Autodesk Fusion 360 part; units mm, degrees
(part 4 of 5)
  spline S14 degree 5 poles (-118.7463, -28.9627) (-118.7429, -28.9568) (-118.7364, -28.9449) (-118.7271, -28.9268) (-118.7157, -28.9022) (-118.7027, -28.8708) (-118.6906, -28.8389) (-118.6791, -28.8067) (-118.668, -28.7744) (-118.657, -28.7419) (-118.6463, -28.7093) (-118.6358, -28.6766) (-118.6257, -28.6437) (-118.6161, -28.6105) (-118.607, -28.5772) (-118.5983, -28.5436) (-118.59, -28.5099) (-118.582, -28.476) (-118.5742, -28.4421) (-118.5667, -28.408) (-118.5595, -28.3737) (-118.5526, -28.3394) (-118.5459, -28.305) (-118.5395, -28.2704) (-118.5334, -28.2357) (-118.5276, -28.2008) (-118.5221, -28.1659) (-118.5168, -28.1309) (-118.5118, -28.0957) (-118.507, -28.0605) (-118.5025, -28.0252) (-118.4982, -27.9897) (-118.4942, -27.9542) (-118.4904, -27.9186) (-118.4868, -27.8829) (-118.4835, -27.8471) (-118.4804, -27.8113) (-118.4775, -27.7753) (-118.4749, -27.7393) (-118.4725, -27.7032) (-118.4703, -27.667) (-118.4684, -27.6307) (-118.4666, -27.5944) (-118.4651, -27.558) (-118.4638, -27.5215) (-118.4627, -27.4849) (-118.4618, -27.4483) (-118.4612, -27.4116) (-118.4607, -27.3749) (-118.4605, -27.3381) (-118.4604, -27.3012) (-118.4606, -27.2643) (-118.461, -27.2273) (-118.4616, -27.1902) (-118.4624, -27.1531) (-118.4634, -27.1159) (-118.4646, -27.0787) (-118.466, -27.0414) (-118.4676, -27.0041) (-118.4694, -26.9667) (-118.4714, -26.9293) (-118.4736, -26.8918) (-118.476, -26.8542) (-118.4785, -26.8167) (-118.4813, -26.779) (-118.4843, -26.7414) (-118.4875, -26.7036) (-118.4908, -26.6659) (-118.4944, -26.6281) (-118.4981, -26.5902) (-118.5021, -26.5523) (-118.5053, -26.522) (-118.5079, -26.4992) (-118.5097, -26.484) (-118.5105, -26.4764) knots 0 0 0 0 0 0 0.01428571 0.02857143 0.04285714 0.05714286 0.07142857 0.08571429 0.1 0.11428571 0.12857143 0.14285714 0.15714286 0.17142857 0.18571429 0.2 0.21428571 0.22857143 0.24285714 0.25714286 0.27142857 0.28571429 0.3 0.31428571 0.32857143 0.34285714 0.35714286 0.37142857 0.38571429 0.4 0.41428571 0.42857143 0.44285714 0.45714286 0.47142857 0.48571429 0.5 0.51428571 0.52857143 0.54285714 0.55714286 0.57142857 0.58571429 0.6 0.61428571 0.62857143 0.64285714 0.65714286 0.67142857 0.68571429 0.7 0.71428571 0.72857143 0.74285714 0.75714286 0.77142857 0.78571429 0.8 0.81428571 0.82857143 0.84285714 0.85714286 0.87142857 0.88571429 0.9 0.91428571 0.92857143 0.94285714 0.95714286 0.97142857 0.98571429 1 1 1 1 1 1
  arc A29 (-118.5105, -26.4764) -> (-119.3694, -26.0969) centre (-125, -40) ccw
  spline S15 degree 5 poles (-121.0491, -27.9451) (-121.047, -27.9386) (-121.0426, -27.9258) (-121.0354, -27.9067) (-121.025, -27.8817) (-121.0105, -27.8509) (-120.995, -27.8206) (-120.979, -27.7904) (-120.9626, -27.7604) (-120.9459, -27.7304) (-120.9291, -27.7005) (-120.9119, -27.6708) (-120.8943, -27.6412) (-120.8763, -27.6118) (-120.8578, -27.5825) (-120.8388, -27.5535) (-120.8195, -27.5247) (-120.7999, -27.4959) (-120.78, -27.4673) (-120.7598, -27.4388) (-120.7393, -27.4105) (-120.7186, -27.3822) (-120.6977, -27.3541) (-120.6764, -27.3261) (-120.6548, -27.2982) (-120.633, -27.2705) (-120.6109, -27.2429) (-120.5885, -27.2154) (-120.5659, -27.188) (-120.543, -27.1608) (-120.52, -27.1336) (-120.4967, -27.1066) (-120.4731, -27.0797) (-120.4494, -27.0529) (-120.4254, -27.0263) (-120.4011, -26.9997) (-120.3767, -26.9733) (-120.352, -26.947) (-120.3272, -26.9208) (-120.3021, -26.8947) (-120.2768, -26.8687) (-120.2513, -26.8428) (-120.2256, -26.8171) (-120.1997, -26.7914) (-120.1736, -26.7659) (-120.1473, -26.7405) (-120.1208, -26.7152) (-120.0942, -26.69) (-120.0673, -26.6649) (-120.0402, -26.64) (-120.013, -26.6151) (-119.9856, -26.5904) (-119.9579, -26.5658) (-119.9301, -26.5412) (-119.9022, -26.5168) (-119.874, -26.4926) (-119.8457, -26.4684) (-119.8172, -26.4443) (-119.7885, -26.4204) (-119.7596, -26.3965) (-119.7306, -26.3728) (-119.7014, -26.3492) (-119.6721, -26.3257) (-119.6425, -26.3023) (-119.6128, -26.279) (-119.583, -26.2558) (-119.553, -26.2328) (-119.5228, -26.2099) (-119.4924, -26.187) (-119.4619, -26.1643) (-119.4313, -26.1417) (-119.4066, -26.1237) (-119.388, -26.1103) (-119.3756, -26.1014) (-119.3694, -26.0969) knots 0 0 0 0 0 0 0.01428571 0.02857143 0.04285714 0.05714286 0.07142857 0.08571429 0.1 0.11428571 0.12857143 0.14285714 0.15714286 0.17142857 0.18571429 0.2 0.21428571 0.22857143 0.24285714 0.25714286 0.27142857 0.28571429 0.3 0.31428571 0.32857143 0.34285714 0.35714286 0.37142857 0.38571429 0.4 0.41428571 0.42857143 0.44285714 0.45714286 0.47142857 0.48571429 0.5 0.51428571 0.52857143 0.54285714 0.55714286 0.57142857 0.58571429 0.6 0.61428571 0.62857143 0.64285714 0.65714286 0.67142857 0.68571429 0.7 0.71428571 0.72857143 0.74285714 0.75714286 0.77142857 0.78571429 0.8 0.81428571 0.82857143 0.84285714 0.85714286 0.87142857 0.88571429 0.9 0.91428571 0.92857143 0.94285714 0.95714286 0.97142857 0.98571429 1 1 1 1 1 1
  line L15 (-121.0491, -27.9451) -> (-121.1835, -28.3552)
  arc A30 (-121.7948, -28.6805) -> (-121.1835, -28.3552) centre (-121.6586, -28.1994) ccw
  arc A31 (-121.7948, -28.6805) -> (-122.5797, -28.4872) centre (-125, -40) ccw
  arc A32 (-122.9699, -27.915) -> (-122.5797, -28.4872) centre (-122.4768, -27.9979) ccw
  line L16 (-122.9699, -27.915) -> (-122.8984, -27.4894)
  spline S16 degree 5 poles (-122.8984, -27.4894) (-122.8973, -27.4827) (-122.8952, -27.4693) (-122.8927, -27.4491) (-122.8903, -27.4221) (-122.8889, -27.3881) (-122.8884, -27.3541) (-122.8887, -27.3199) (-122.8892, -27.2857) (-122.89, -27.2514) (-122.8911, -27.2171) (-122.8924, -27.1828) (-122.8943, -27.1484) (-122.8966, -27.114) (-122.8994, -27.0795) (-122.9027, -27.045) (-122.9064, -27.0105) (-122.9104, -26.9759) (-122.9148, -26.9413) (-122.9194, -26.9067) (-122.9243, -26.8721) (-122.9295, -26.8375) (-122.9351, -26.8028) (-122.9409, -26.7681) (-122.9471, -26.7334) (-122.9535, -26.6987) (-122.9603, -26.664) (-122.9673, -26.6293) (-122.9746, -26.5946) (-122.9822, -26.5598) (-122.99, -26.5251) (-122.9981, -26.4903) (-123.0064, -26.4556) (-123.015, -26.4208) (-123.0239, -26.386) (-123.033, -26.3513) (-123.0424, -26.3165) (-123.052, -26.2817) (-123.0618, -26.247) (-123.0719, -26.2122) (-123.0822, -26.1775) (-123.0928, -26.1427) (-123.1036, -26.108) (-123.1146, -26.0733) (-123.1259, -26.0385) (-123.1373, -26.0038) (-123.1491, -25.9691) (-123.161, -25.9344) (-123.1731, -25.8997) (-123.1855, -25.865) (-123.1981, -25.8304) (-123.2109, -25.7957) (-123.2239, -25.7611) (-123.2371, -25.7265) (-123.2506, -25.6919) (-123.2642, -25.6573) (-123.2781, -25.6227) (-123.2921, -25.5882) (-123.3064, -25.5536) (-123.3209, -25.5191) (-123.3356, -25.4846) (-123.3504, -25.4501) (-123.3655, -25.4157) (-123.3808, -25.3812) (-123.3963, -25.3468) (-123.412, -25.3125) (-123.4278, -25.2781) (-123.4439, -25.2438) (-123.4602, -25.2094) (-123.4766, -25.1752) (-123.4933, -25.1409) (-123.5068, -25.1135) (-123.517, -25.093) (-123.5238, -25.0793) (-123.5272, -25.0725) knots 0 0 0 0 0 0 0.01428571 0.02857143 0.04285714 0.05714286 0.07142857 0.08571429 0.1 0.11428571 0.12857143 0.14285714 0.15714286 0.17142857 0.18571429 0.2 0.21428571 0.22857143 0.24285714 0.25714286 0.27142857 0.28571429 0.3 0.31428571 0.32857143 0.34285714 0.35714286 0.37142857 0.38571429 0.4 0.41428571 0.42857143 0.44285714 0.45714286 0.47142857 0.48571429 0.5 0.51428571 0.52857143 0.54285714 0.55714286 0.57142857 0.58571429 0.6 0.61428571 0.62857143 0.64285714 0.65714286 0.67142857 0.68571429 0.7 0.71428571 0.72857143 0.74285714 0.75714286 0.77142857 0.78571429 0.8 0.81428571 0.82857143 0.84285714 0.85714286 0.87142857 0.88571429 0.9 0.91428571 0.92857143 0.94285714 0.95714286 0.97142857 0.98571429 1 1 1 1 1 1
  arc A33 (-123.5272, -25.0725) -> (-124.4641, -25.0096) centre (-125, -40) ccw
  spline S17 degree 5 poles (-125.4104, -27.3208) (-125.4106, -27.314) (-125.4109, -27.3004) (-125.4107, -27.2801) (-125.4094, -27.253) (-125.4063, -27.2191) (-125.4022, -27.1853) (-125.3974, -27.1515) (-125.3923, -27.1176) (-125.3869, -27.0838) (-125.3813, -27.0499) (-125.3753, -27.0161) (-125.3689, -26.9823) (-125.362, -26.9485) (-125.3546, -26.9147) (-125.3467, -26.8809) (-125.3385, -26.8472) (-125.3298, -26.8135) (-125.3209, -26.7798) (-125.3117, -26.7461) (-125.3022, -26.7125) (-125.2924, -26.6788) (-125.2823, -26.6452) (-125.2719, -26.6116) (-125.2611, -26.5781) (-125.2501, -26.5446) (-125.2387, -26.511) (-125.2271, -26.4776) (-125.2153, -26.4441) (-125.2031, -26.4107) (-125.1907, -26.3773) (-125.1781, -26.344) (-125.1651, -26.3106) (-125.152, -26.2773) (-125.1385, -26.2441) (-125.1249, -26.2108) (-125.1109, -26.1776) (-125.0968, -26.1445) (-125.0823, -26.1113) (-125.0677, -26.0782) (-125.0528, -26.0452) (-125.0377, -26.0121) (-125.0224, -25.9792) (-125.0068, -25.9462) (-124.991, -25.9133) (-124.975, -25.8804) (-124.9588, -25.8476) (-124.9423, -25.8148) (-124.9256, -25.7821) (-124.9087, -25.7493) (-124.8916, -25.7167) (-124.8743, -25.684) (-124.8568, -25.6515) (-124.8391, -25.6189) (-124.8211, -25.5864) (-124.803, -25.554) (-124.7846, -25.5216) (-124.7661, -25.4892) (-124.7473, -25.4569) (-124.7283, -25.4246) (-124.7092, -25.3924) (-124.6898, -25.3602) (-124.6703, -25.3281) (-124.6505, -25.296) (-124.6306, -25.264) (-124.6104, -25.232) (-124.5901, -25.2001) (-124.5696, -25.1682) (-124.5489, -25.1364) (-124.528, -25.1046) (-124.5069, -25.0729) (-124.4899, -25.0475) (-124.477, -25.0285) (-124.4684, -25.0159) (-124.4641, -25.0096) knots 0 0 0 0 0 0 0.01428571 0.02857143 0.04285714 0.05714286 0.07142857 0.08571429 0.1 0.11428571 0.12857143 0.14285714 0.15714286 0.17142857 0.18571429 0.2 0.21428571 0.22857143 0.24285714 0.25714286 0.27142857 0.28571429 0.3 0.31428571 0.32857143 0.34285714 0.35714286 0.37142857 0.38571429 0.4 0.41428571 0.42857143 0.44285714 0.45714286 0.47142857 0.48571429 0.5 0.51428571 0.52857143 0.54285714 0.55714286 0.57142857 0.58571429 0.6 0.61428571 0.62857143 0.64285714 0.65714286 0.67142857 0.68571429 0.7 0.71428571 0.72857143 0.74285714 0.75714286 0.77142857 0.78571429 0.8 0.81428571 0.82857143 0.84285714 0.85714286 0.87142857 0.88571429 0.9 0.91428571 0.92857143 0.94285714 0.95714286 0.97142857 0.98571429 1 1 1 1 1 1
  line L17 (-125.4104, -27.3208) -> (-125.3964, -27.7521)
  arc A34 (-125.8596, -28.2669) -> (-125.3964, -27.7521) centre (-125.8962, -27.7683) ccw
  arc A35 (-125.8596, -28.2669) -> (-126.6633, -28.3537) centre (-125, -40) ccw
  arc A36 (-127.2256, -27.9495) -> (-126.6633, -28.3537) centre (-126.734, -27.8587) ccw
  line L18 (-127.2256, -27.9495) -> (-127.304, -27.5251)
  spline S18 degree 5 poles (-127.304, -27.5251) (-127.3053, -27.5185) (-127.3079, -27.5051) (-127.3124, -27.4853) (-127.3195, -27.4591) (-127.3297, -27.4267) (-127.3409, -27.3945) (-127.3528, -27.3625) (-127.3651, -27.3305) (-127.3775, -27.2986) (-127.3903, -27.2667) (-127.4033, -27.2349) (-127.4167, -27.2033) (-127.4307, -27.1717) (-127.4451, -27.1403) (-127.46, -27.109) (-127.4753, -27.0778) (-127.491, -27.0467) (-127.5069, -27.0157) (-127.5231, -26.9848) (-127.5395, -26.9539) (-127.5563, -26.9231) (-127.5733, -26.8924) (-127.5906, -26.8619) (-127.6083, -26.8314) (-127.6262, -26.801) (-127.6445, -26.7707) (-127.6629, -26.7404) (-127.6817, -26.7103) (-127.7007, -26.6802) (-127.7199, -26.6502) (-127.7394, -26.6203) (-127.7591, -26.5905) (-127.7791, -26.5608) (-127.7993, -26.5312) (-127.8198, -26.5016) (-127.8405, -26.4722) (-127.8614, -26.4428) (-127.8825, -26.4135) (-127.9039, -26.3843) (-127.9255, -26.3552) (-127.9473, -26.3261) (-127.9693, -26.2972) (-127.9915, -26.2683) (-128.014, -26.2395) (-128.0367, -26.2108) (-128.0595, -26.1822) (-128.0826, -26.1537) (-128.1059, -26.1252) (-128.1294, -26.0969) (-128.153, -26.0686) (-128.1769, -26.0404) (-128.201, -26.0123) (-128.2253, -25.9843) (-128.2497, -25.9564) (-128.2744, -25.9286) (-128.2992, -25.9008) (-128.3243, -25.8732) (-128.3495, -25.8456) (-128.3749, -25.8181) (-128.4005, -25.7907) (-128.4263, -25.7634) (-128.4522, -25.7362) (-128.4784, -25.7091) (-128.5047, -25.682) (-128.5312, -25.6551) (-128.5578, -25.6282) (-128.5847, -25.6015) (-128.6117, -25.5748) (-128.6389, -25.5482) (-128.6663, -25.5217) (-128.6883, -25.5006) (-128.7049, -25.4848) (-128.716, -25.4743) (-128.7216, -25.469) knots 0 0 0 0 0 0 0.01428571 0.02857143 0.04285714 0.05714286 0.07142857 0.08571429 0.1 0.11428571 0.12857143 0.14285714 0.15714286 0.17142857 0.18571429 0.2 0.21428571 0.22857143 0.24285714 0.25714286 0.27142857 0.28571429 0.3 0.31428571 0.32857143 0.34285714 0.35714286 0.37142857 0.38571429 0.4 0.41428571 0.42857143 0.44285714 0.45714286 0.47142857 0.48571429 0.5 0.51428571 0.52857143 0.54285714 0.55714286 0.57142857 0.58571429 0.6 0.61428571 0.62857143 0.64285714 0.65714286 0.67142857 0.68571429 0.7 0.71428571 0.72857143 0.74285714 0.75714286 0.77142857 0.78571429 0.8 0.81428571 0.82857143 0.84285714 0.85714286 0.87142857 0.88571429 0.9 0.91428571 0.92857143 0.94285714 0.95714286 0.97142857 0.98571429 1 1 1 1 1 1
  arc A37 (-128.7216, -25.469) -> (-129.6235, -25.7303) centre (-125, -40) ccw
  spline S19 degree 5 poles (-129.7222, -28.2258) (-129.7247, -28.2195) (-129.7296, -28.2068) (-129.7364, -28.1876) (-129.7444, -28.1617) (-129.7531, -28.1289) (-129.7608, -28.0957) (-129.7679, -28.0622) (-129.7746, -28.0287) (-129.7812, -27.995) (-129.7874, -27.9613) (-129.7934, -27.9275) (-129.799, -27.8935) (-129.8041, -27.8594) (-129.8087, -27.8251) (-129.8128, -27.7907) (-129.8166, -27.7562) (-129.82, -27.7215) (-129.8231, -27.6868) (-129.826, -27.652) (-129.8286, -27.6172) (-129.8309, -27.5822) (-129.8329, -27.5472) (-129.8346, -27.512) (-129.8359, -27.4768) (-129.837, -27.4415) (-129.8378, -27.4062) (-129.8384, -27.3708) (-129.8387, -27.3353) (-129.8387, -27.2997) (-129.8384, -27.2641) (-129.838, -27.2284) (-129.8372, -27.1927) (-129.8362, -27.1569) (-129.835, -27.121) (-129.8335, -27.0851) (-129.8318, -27.0492) (-129.8298, -27.0131) (-129.8276, -26.9771) (-129.8251, -26.941) (-129.8225, -26.9048) (-129.8196, -26.8686) (-129.8164, -26.8324) (-129.8131, -26.7961) (-129.8095, -26.7598) (-129.8057, -26.7234) (-129.8017, -26.687) (-129.7974, -26.6505) (-129.7929, -26.6141) (-129.7883, -26.5776) (-129.7834, -26.541) (-129.7782, -26.5044) (-129.7729, -26.4678) (-129.7674, -26.4312) (-129.7616, -26.3945) (-129.7557, -26.3578) (-129.7495, -26.321) (-129.7431, -26.2843) (-129.7366, -26.2475) (-129.7298, -26.2107) (-129.7228, -26.1739) (-129.7156, -26.137) (-129.7082, -26.1001) (-129.7007, -26.0632) (-129.6929, -26.0263) (-129.6849, -25.9894) (-129.6767, -25.9524) (-129.6683, -25.9154) (-129.6598, -25.8785) (-129.651, -25.8414) (-129.642, -25.8044) (-129.6347, -25.7748) (-129.6291, -25.7526) (-129.6254, -25.7377) (-129.6235, -25.7303) knots 0 0 0 0 0 0 0.01428571 0.02857143 0.04285714 0.05714286 0.07142857 0.08571429 0.1 0.11428571 0.12857143 0.14285714 0.15714286 0.17142857 0.18571429 0.2 0.21428571 0.22857143 0.24285714 0.25714286 0.27142857 0.28571429 0.3 0.31428571 0.32857143 0.34285714 0.35714286 0.37142857 0.38571429 0.4 0.41428571 0.42857143 0.44285714 0.45714286 0.47142857 0.48571429 0.5 0.51428571 0.52857143 0.54285714 0.55714286 0.57142857 0.58571429 0.6 0.61428571 0.62857143 0.64285714 0.65714286 0.67142857 0.68571429 0.7 0.71428571 0.72857143 0.74285714 0.75714286 0.77142857 0.78571429 0.8 0.81428571 0.82857143 0.84285714 0.85714286 0.87142857 0.88571429 0.9 0.91428571 0.92857143 0.94285714 0.95714286 0.97142857 0.98571429 1 1 1 1 1 1
  line L19 (-129.7222, -28.2258) -> (-129.5615, -28.6263)
  arc A38 (-129.8207, -29.2685) -> (-129.5615, -28.6263) centre (-130.0256, -28.8125) ccw
  arc A39 (-129.8207, -29.2685) -> (-130.5462, -29.6249) centre (-125, -40) ccw
  arc A40 (-131.2129, -29.4375) -> (-130.5462, -29.6249) centre (-130.782, -29.184) ccw
  line L20 (-131.2129, -29.4375) -> (-131.4317, -29.0655)
  spline S20 degree 5 poles (-131.4317, -29.0655) (-131.4352, -29.0596) (-131.4422, -29.048) (-131.4532, -29.0309) (-131.4688, -29.0087) (-131.4895, -28.9817) (-131.5111, -28.9554) (-131.5332, -28.9293) (-131.5557, -28.9035) (-131.5783, -28.8777) (-131.6011, -28.8522) (-131.6243, -28.8267) (-131.6477, -28.8016) (-131.6716, -28.7767) (-131.696, -28.7521) (-131.7207, -28.7278) (-131.7457, -28.7037) (-131.771, -28.6798) (-131.7966, -28.6561) (-131.8224, -28.6326) (-131.8484, -28.6092) (-131.8746, -28.5861) (-131.9011, -28.563) (-131.9279, -28.5402) (-131.9549, -28.5176) (-131.9822, -28.4952) (-132.0097, -28.4729) (-132.0374, -28.4509) (-132.0653, -28.4289) (-132.0934, -28.4072) (-132.1218, -28.3856) (-132.1503, -28.3642) (-132.179, -28.3429) (-132.208, -28.3218) (-132.2371, -28.3009) (-132.2664, -28.2801) (-132.296, -28.2595) (-132.3257, -28.239) (-132.3555, -28.2187) (-132.3856, -28.1986) (-132.4159, -28.1786) (-132.4463, -28.1588) (-132.4769, -28.1391) (-132.5077, -28.1196) (-132.5386, -28.1002) (-132.5697, -28.081) (-132.601, -28.0619) (-132.6324, -28.043) (-132.664, -28.0243) (-132.6958, -28.0056) (-132.7277, -27.9872) (-132.7598, -27.9689) (-132.792, -27.9507) (-132.8244, -27.9327) (-132.8569, -27.9148) (-132.8896, -27.8971) (-132.9225, -27.8795) (-132.9554, -27.8621) (-132.9886, -27.8448) (-133.0219, -27.8277) (-133.0553, -27.8107) (-133.0888, -27.7938) (-133.1225, -27.7771) (-133.1564, -27.7606) (-133.1904, -27.7442) (-133.2245, -27.7279) (-133.2587, -27.7118) (-133.2931, -27.6958) (-133.3276, -27.68) (-133.3623, -27.6643) (-133.397, -27.6488) (-133.425, -27.6365) (-133.446, -27.6273) (-133.46, -27.6212) (-133.467, -27.6182) knots 0 0 0 0 0 0 0.01428571 0.02857143 0.04285714 0.05714286 0.07142857 0.08571429 0.1 0.11428571 0.12857143 0.14285714 0.15714286 0.17142857 0.18571429 0.2 0.21428571 0.22857143 0.24285714 0.25714286 0.27142857 0.28571429 0.3 0.31428571 0.32857143 0.34285714 0.35714286 0.37142857 0.38571429 0.4 0.41428571 0.42857143 0.44285714 0.45714286 0.47142857 0.48571429 0.5 0.51428571 0.52857143 0.54285714 0.55714286 0.57142857 0.58571429 0.6 0.61428571 0.62857143 0.64285714 0.65714286 0.67142857 0.68571429 0.7 0.71428571 0.72857143 0.74285714 0.75714286 0.77142857 0.78571429 0.8 0.81428571 0.82857143 0.84285714 0.85714286 0.87142857 0.88571429 0.9 0.91428571 0.92857143 0.94285714 0.95714286 0.97142857 0.98571429 1 1 1 1 1 1
  arc A41 (-133.467, -27.6182) -> (-134.2252, -28.1722) centre (-125, -40) ccw
  spline S21 degree 5 poles (-133.4644, -30.5509) (-133.4689, -30.5459) (-133.4779, -30.5357) (-133.4908, -30.52) (-133.5072, -30.4984) (-133.5266, -30.4704) (-133.5452, -30.4419) (-133.5633, -30.4129) (-133.5811, -30.3837) (-133.5988, -30.3543) (-133.6162, -30.3247) (-133.6334, -30.295) (-133.6502, -30.265) (-133.6667, -30.2347) (-133.6827, -30.204) (-133.6984, -30.1731) (-133.7137, -30.1419) (-133.7288, -30.1106) (-133.7436, -30.079) (-133.7582, -30.0473) (-133.7725, -30.0154) (-133.7867, -29.9833) (-133.8005, -29.9511) (-133.8141, -29.9187) (-133.8275, -29.8861) (-133.8406, -29.8533) (-133.8534, -29.8203) (-133.866, -29.7872) (-133.8784, -29.754) (-133.8906, -29.7206) (-133.9026, -29.687) (-133.9143, -29.6533) (-133.9259, -29.6195) (-133.9372, -29.5855) (-133.9483, -29.5514) (-133.9592, -29.5171) (-133.9698, -29.4827) (-133.9803, -29.4482) (-133.9905, -29.4136) (-134.0006, -29.3788) (-134.0105, -29.3439) (-134.0201, -29.3089) (-134.0296, -29.2738) (-134.0388, -29.2386) (-134.0479, -29.2032) (-134.0567, -29.1677) (-134.0654, -29.1321) (-134.0739, -29.0964) (-134.0822, -29.0606) (-134.0902, -29.0247) (-134.0981, -28.9887) (-134.1058, -28.9526) (-134.1134, -28.9163) (-134.1207, -28.88) (-134.1278, -28.8436) (-134.1348, -28.807) (-134.1416, -28.7704) (-134.1482, -28.7337) (-134.1546, -28.6969) (-134.1608, -28.66) (-134.1668, -28.623) (-134.1727, -28.5859) (-134.1783, -28.5487) (-134.1838, -28.5114) (-134.1891, -28.4741) (-134.1943, -28.4366) (-134.1992, -28.3991) (-134.204, -28.3615) (-134.2086, -28.3238) (-134.213, -28.286) (-134.2173, -28.2482) (-134.2205, -28.2178) (-134.2229, -28.195) (-134.2244, -28.1798) (-134.2252, -28.1722) knots 0 0 0 0 0 0 0.01428571 0.02857143 0.04285714 0.05714286 0.07142857 0.08571429 0.1 0.11428571 0.12857143 0.14285714 0.15714286 0.17142857 0.18571429 0.2 0.21428571 0.22857143 0.24285714 0.25714286 0.27142857 0.28571429 0.3 0.31428571 0.32857143 0.34285714 0.35714286 0.37142857 0.38571429 0.4 0.41428571 0.42857143 0.44285714 0.45714286 0.47142857 0.48571429 0.5 0.51428571 0.52857143 0.54285714 0.55714286 0.57142857 0.58571429 0.6 0.61428571 0.62857143 0.64285714 0.65714286 0.67142857 0.68571429 0.7 0.71428571 0.72857143 0.74285714 0.75714286 0.77142857 0.78571429 0.8 0.81428571 0.82857143 0.84285714 0.85714286 0.87142857 0.88571429 0.9 0.91428571 0.92857143 0.94285714 0.95714286 0.97142857 0.98571429 1 1 1 1 1 1
  line L21 (-133.4644, -30.5509) -> (-133.1765, -30.8724)
  arc A42 (-133.2004, -31.5645) -> (-133.1765, -30.8724) centre (-133.5489, -31.206) ccw
  arc A43 (-133.2004, -31.5645) -> (-133.7603, -32.1475) centre (-125, -40) ccw
  arc A44 (-134.4509, -32.1994) -> (-133.7603, -32.1475) centre (-134.1326, -31.8138) ccw
  line L22 (-134.4509, -32.1994) -> (-134.7837, -31.9247)
  spline S22 degree 5 poles (-134.7837, -31.9247) (-134.7889, -31.9204) (-134.7995, -31.9119) (-134.8157, -31.8996) (-134.838, -31.884) (-134.8666, -31.8658) (-134.8959, -31.8484) (-134.9256, -31.8315) (-134.9555, -31.8148) (-134.9856, -31.7984) (-135.0158, -31.7822) (-135.0463, -31.7662) (-135.0769, -31.7506) (-135.1079, -31.7354) (-135.1391, -31.7206) (-135.1707, -31.7062) (-135.2024, -31.6921) (-135.2344, -31.6784) (-135.2665, -31.6648) (-135.2988, -31.6515) (-135.3313, -31.6385) (-135.3639, -31.6257) (-135.3966, -31.6131) (-135.4296, -31.6008) (-135.4627, -31.5888) (-135.496, -31.5771) (-135.5294, -31.5656) (-135.563, -31.5543) (-135.5968, -31.5432) (-135.6306, -31.5324) (-135.6646, -31.5218) (-135.6988, -31.5114) (-135.733, -31.5013) (-135.7675, -31.4914) (-135.802, -31.4817) (-135.8367, -31.4722) (-135.8714, -31.4629) (-135.9064, -31.4538) (-135.9414, -31.445) (-135.9765, -31.4363) (-136.0118, -31.4279) (-136.0472, -31.4197) (-136.0826, -31.4117) (-136.1182, -31.4038) (-136.1539, -31.3962) (-136.1897, -31.3888) (-136.2256, -31.3816) (-136.2617, -31.3746) (-136.2978, -31.3677) (-136.334, -31.3611) (-136.3703, -31.3547) (-136.4067, -31.3484) (-136.4432, -31.3424) (-136.4798, -31.3365) (-136.5165, -31.3309) (-136.5533, -31.3254) (-136.5901, -31.3201) (-136.6271, -31.315) (-136.6641, -31.3101) (-136.7013, -31.3054) (-136.7385, -31.3008) (-136.7758, -31.2965) (-136.8131, -31.2923) (-136.8506, -31.2884) (-136.8881, -31.2846) (-136.9258, -31.2809) (-136.9635, -31.2775) (-137.0012, -31.2743) (-137.0391, -31.2712) (-137.077, -31.2683) (-137.115, -31.2656) (-137.1455, -31.2636) (-137.1683, -31.2622) (-137.1836, -31.2612) (-137.1912, -31.2608) knots 0 0 0 0 0 0 0.01428571 0.02857143 0.04285714 0.05714286 0.07142857 0.08571429 0.1 0.11428571 0.12857143 0.14285714 0.15714286 0.17142857 0.18571429 0.2 0.21428571 0.22857143 0.24285714 0.25714286 0.27142857 0.28571429 0.3 0.31428571 0.32857143 0.34285714 0.35714286 0.37142857 0.38571429 0.4 0.41428571 0.42857143 0.44285714 0.45714286 0.47142857 0.48571429 0.5 0.51428571 0.52857143 0.54285714 0.55714286 0.57142857 0.58571429 0.6 0.61428571 0.62857143 0.64285714 0.65714286 0.67142857 0.68571429 0.7 0.71428571 0.72857143 0.74285714 0.75714286 0.77142857 0.78571429 0.8 0.81428571 0.82857143 0.84285714 0.85714286 0.87142857 0.88571429 0.9 0.91428571 0.92857143 0.94285714 0.95714286 0.97142857 0.98571429 1 1 1 1 1 1
  arc A45 (-137.1912, -31.2608) -> (-137.7142, -32.0407) centre (-125, -40) ccw
  spline S23 degree 5 poles (-136.1857, -34.0158) (-136.1917, -34.0126) (-136.2036, -34.006) (-136.2211, -33.9957) (-136.2439, -33.981) (-136.2717, -33.9614) (-136.299, -33.9409) (-136.3259, -33.9199) (-136.3526, -33.8985) (-136.3792, -33.8769) (-136.4057, -33.8551) (-136.432, -33.8331) (-136.4581, -33.8106) (-136.484, -33.7878) (-136.5095, -33.7645) (-136.5348, -33.7408) (-136.5599, -33.7167) (-136.5848, -33.6924) (-136.6095, -33.6678) (-136.634, -33.643) (-136.6584, -33.6179) (-136.6827, -33.5926) (-136.7067, -33.5671) (-136.7306, -33.5413) (-136.7543, -33.5152) (-136.7778, -33.4889) (-136.8011, -33.4623) (-136.8243, -33.4355) (-136.8474, -33.4085) (-136.8702, -33.3813) (-136.8929, -33.3538) (-136.9155, -33.3262) (-136.9379, -33.2983) (-136.9602, -33.2703) (-136.9823, -33.242) (-137.0042, -33.2135) (-137.026, -33.1849) (-137.0476, -33.156) (-137.0691, -33.127) (-137.0905, -33.0977) (-137.1116, -33.0683) (-137.1327, -33.0387) (-137.1536, -33.009) (-137.1743, -32.979) (-137.1949, -32.9489) (-137.2154, -32.9186) (-137.2357, -32.8881) (-137.2559, -32.8574) (-137.2759, -32.8266) (-137.2958, -32.7956) (-137.3155, -32.7645) (-137.3351, -32.7332) (-137.3546, -32.7017) (-137.3739, -32.6701) (-137.3931, -32.6383) (-137.4121, -32.6063) (-137.431, -32.5742) (-137.4498, -32.542) (-137.4684, -32.5096) (-137.4868, -32.477) (-137.5052, -32.4443) (-137.5233, -32.4115) (-137.5414, -32.3785) (-137.5593, -32.3453) (-137.5771, -32.3121) (-137.5947, -32.2786) (-137.6122, -32.2451) (-137.6295, -32.2113) (-137.6467, -32.1775) (-137.6638, -32.1435) (-137.6807, -32.1094) (-137.6942, -32.082) (-137.7042, -32.0614) (-137.7108, -32.0476) (-137.7142, -32.0407) knots 0 0 0 0 0 0 0.01428571 0.02857143 0.04285714 0.05714286 0.07142857 0.08571429 0.1 0.11428571 0.12857143 0.14285714 0.15714286 0.17142857 0.18571429 0.2 0.21428571 0.22857143 0.24285714 0.25714286 0.27142857 0.28571429 0.3 0.31428571 0.32857143 0.34285714 0.35714286 0.37142857 0.38571429 0.4 0.41428571 0.42857143 0.44285714 0.45714286 0.47142857 0.48571429 0.5 0.51428571 0.52857143 0.54285714 0.55714286 0.57142857 0.58571429 0.6 0.61428571 0.62857143 0.64285714 0.65714286 0.67142857 0.68571429 0.7 0.71428571 0.72857143 0.74285714 0.75714286 0.77142857 0.78571429 0.8 0.81428571 0.82857143 0.84285714 0.85714286 0.87142857 0.88571429 0.9 0.91428571 0.92857143 0.94285714 0.95714286 0.97142857 0.98571429 1 1 1 1 1 1
  line L23 (-136.1857, -34.0158) -> (-135.8052, -34.2194)
  arc A46 (-135.5909, -34.8779) -> (-135.8052, -34.2194) centre (-136.0411, -34.6602) ccw
  arc A47 (-135.5909, -34.8779) -> (-135.9177, -35.6173) centre (-125, -40) ccw
  arc A48 (-136.5489, -35.9022) -> (-135.9177, -35.6173) centre (-136.3817, -35.431) ccw
  line L24 (-136.5489, -35.9022) -> (-136.9556, -35.7579)
  spline S24 degree 5 poles (-136.9556, -35.7579) (-136.962, -35.7556) (-136.9748, -35.7513) (-136.9943, -35.7453) (-137.0205, -35.7383) (-137.0537, -35.7309) (-137.0872, -35.7246) (-137.1208, -35.7188) (-137.1546, -35.7135) (-137.1885, -35.7083) (-137.2225, -35.7034) (-137.2565, -35.6988) (-137.2907, -35.6946) (-137.325, -35.6909) (-137.3594, -35.6877) (-137.394, -35.6849) (-137.4286, -35.6826) (-137.4634, -35.6806) (-137.4982, -35.6789) (-137.5331, -35.6774) (-137.568, -35.6762) (-137.603, -35.6753) (-137.6381, -35.6748) (-137.6733, -35.6745) (-137.7085, -35.6745) (-137.7438, -35.6749) (-137.7792, -35.6755) (-137.8146, -35.6764) (-137.8501, -35.6775) (-137.8856, -35.679) (-137.9212, -35.6806) (-137.9568, -35.6826) (-137.9925, -35.6847) (-138.0282, -35.6872) (-138.064, -35.6899) (-138.0998, -35.6928) (-138.1357, -35.696) (-138.1716, -35.6994) (-138.2075, -35.7031) (-138.2435, -35.707) (-138.2795, -35.7111) (-138.3156, -35.7155) (-138.3517, -35.7201) (-138.3878, -35.7249) (-138.4239, -35.73) (-138.4601, -35.7352) (-138.4963, -35.7407) (-138.5326, -35.7465) (-138.5688, -35.7524) (-138.6051, -35.7585) (-138.6415, -35.7649) (-138.6778, -35.7715) (-138.7142, -35.7783) (-138.7506, -35.7853) (-138.787, -35.7925) (-138.8234, -35.8) (-138.8599, -35.8076) (-138.8963, -35.8155) (-138.9328, -35.8235) (-138.9693, -35.8318) (-139.0058, -35.8403) (-139.0424, -35.8489) (-139.0789, -35.8578) (-139.1155, -35.8669) (-139.1521, -35.8762) (-139.1886, -35.8856) (-139.2252, -35.8953) (-139.2618, -35.9052) (-139.2985, -35.9152) (-139.3351, -35.9255) (-139.3717, -35.9359) (-139.401, -35.9444) (-139.423, -35.9509) (-139.4377, -35.9553) (-139.445, -35.9575) knots 0 0 0 0 0 0 0.01428571 0.02857143 0.04285714 0.05714286 0.07142857 0.08571429 0.1 0.11428571 0.12857143 0.14285714 0.15714286 0.17142857 0.18571429 0.2 0.21428571 0.22857143 0.24285714 0.25714286 0.27142857 0.28571429 0.3 0.31428571 0.32857143 0.34285714 0.35714286 0.37142857 0.38571429 0.4 0.41428571 0.42857143 0.44285714 0.45714286 0.47142857 0.48571429 0.5 0.51428571 0.52857143 0.54285714 0.55714286 0.57142857 0.58571429 0.6 0.61428571 0.62857143 0.64285714 0.65714286 0.67142857 0.68571429 0.7 0.71428571 0.72857143 0.74285714 0.75714286 0.77142857 0.78571429 0.8 0.81428571 0.82857143 0.84285714 0.85714286 0.87142857 0.88571429 0.9 0.91428571 0.92857143 0.94285714 0.95714286 0.97142857 0.98571429 1 1 1 1 1 1
  arc A49 (-139.445, -35.9575) -> (-139.6696, -36.8692) centre (-125, -40) ccw
  spline S25 degree 5 poles (-137.5578, -38.2024) (-137.5646, -38.2015) (-137.578, -38.1994) (-137.598, -38.1956) (-137.6245, -38.1897) (-137.6573, -38.1808) (-137.6899, -38.1708) (-137.7224, -38.1602) (-137.7548, -38.1493) (-137.7872, -38.1381) (-137.8195, -38.1267) (-137.8518, -38.115) (-137.884, -38.1028) (-137.9161, -38.0902) (-137.9481, -38.077) (-137.98, -38.0634) (-138.0117, -38.0494) (-138.0434, -38.035) (-138.0751, -38.0203) (-138.1066, -38.0054) (-138.1381, -37.9902) (-138.1696, -37.9747) (-138.2009, -37.959) (-138.2322, -37.9429) (-138.2634, -37.9265) (-138.2945, -37.9098) (-138.3255, -37.8928) (-138.3564, -37.8755) (-138.3873, -37.858) (-138.4181, -37.8403) (-138.4488, -37.8223) (-138.4795, -37.804) (-138.5101, -37.7855) (-138.5406, -37.7667) (-138.571, -37.7477) (-138.6014, -37.7285) (-138.6316, -37.709) (-138.6618, -37.6893) (-138.692, -37.6694) (-138.722, -37.6492) (-138.752, -37.6288) (-138.7819, -37.6082) (-138.8117, -37.5873) (-138.8415, -37.5663) (-138.8711, -37.545) (-138.9007, -37.5235) (-138.9302, -37.5019) (-138.9597, -37.48) (-138.989, -37.4578) (-139.0183, -37.4355) (-139.0475, -37.413) (-139.0766, -37.3903) (-139.1057, -37.3674) (-139.1347, -37.3443) (-139.1635, -37.3209) (-139.1923, -37.2974) (-139.2211, -37.2737) (-139.2497, -37.2498) (-139.2783, -37.2257) (-139.3068, -37.2015) (-139.3352, -37.177) (-139.3635, -37.1524) (-139.3918, -37.1275) (-139.4199, -37.1025) (-139.448, -37.0773) (-139.476, -37.0519) (-139.5039, -37.0264) (-139.5317, -37.0006) (-139.5595, -36.9747) (-139.5872, -36.9486) (-139.6147, -36.9223) (-139.6367, -36.9012) (-139.6532, -36.8852) (-139.6642, -36.8746) (-139.6696, -36.8692) knots 0 0 0 0 0 0 0.01428571 0.02857143 0.04285714 0.05714286 0.07142857 0.08571429 0.1 0.11428571 0.12857143 0.14285714 0.15714286 0.17142857 0.18571429 0.2 0.21428571 0.22857143 0.24285714 0.25714286 0.27142857 0.28571429 0.3 0.31428571 0.32857143 0.34285714 0.35714286 0.37142857 0.38571429 0.4 0.41428571 0.42857143 0.44285714 0.45714286 0.47142857 0.48571429 0.5 0.51428571 0.52857143 0.54285714 0.55714286 0.57142857 0.58571429 0.6 0.61428571 0.62857143 0.64285714 0.65714286 0.67142857 0.68571429 0.7 0.71428571 0.72857143 0.74285714 0.75714286 0.77142857 0.78571429 0.8 0.81428571 0.82857143 0.84285714 0.85714286 0.87142857 0.88571429 0.9 0.91428571 0.92857143 0.94285714 0.95714286 0.97142857 0.98571429 1 1 1 1 1 1
  line L25 (-137.5578, -38.2024) -> (-137.1307, -38.2636)
  arc A50 (-136.7041, -38.8091) -> (-137.1307, -38.2636) centre (-137.2015, -38.7585) ccw
  arc A51 (-136.7041, -38.8091) -> (-136.7582, -39.6156) centre (-125, -40) ccw
  arc A52 (-137.2539, -40.0993) -> (-136.7582, -39.6156) centre (-137.258, -39.5993) ccw
  line L26 (-137.2539, -40.0993) -> (-137.6854, -40.1028)
  spline S26 degree 5 poles (-137.6854, -40.1028) (-137.6922, -40.1028) (-137.7058, -40.1031) (-137.7261, -40.1041) (-137.7532, -40.1065) (-137.7869, -40.111) (-137.8205, -40.1165) (-137.8541, -40.1226) (-137.8877, -40.1291) (-137.9213, -40.1358) (-137.9549, -40.1428) (-137.9885, -40.1502) (-138.022, -40.1579) (-138.0555, -40.1662) (-138.0889, -40.1749) (-138.1223, -40.1842) (-138.1557, -40.1938) (-138.1891, -40.2038) (-138.2224, -40.2141) (-138.2556, -40.2247) (-138.2889, -40.2355) (-138.3221, -40.2466) (-138.3553, -40.2581) (-138.3884, -40.2699) (-138.4215, -40.282) (-138.4546, -40.2943) (-138.4876, -40.307) (-138.5205, -40.32) (-138.5535, -40.3332) (-138.5864, -40.3467) (-138.6193, -40.3604) (-138.6521, -40.3744) (-138.6849, -40.3887) (-138.7176, -40.4032) (-138.7503, -40.418) (-138.7829, -40.433) (-138.8156, -40.4482) (-138.8481, -40.4637) (-138.8806, -40.4795) (-138.9131, -40.4954) (-138.9455, -40.5116) (-138.9779, -40.5281) (-139.0103, -40.5447) (-139.0426, -40.5616) (-139.0748, -40.5787) (-139.107, -40.5961) (-139.1392, -40.6136) (-139.1713, -40.6314) (-139.2033, -40.6494) (-139.2353, -40.6676) (-139.2673, -40.686) (-139.2992, -40.7046) (-139.331, -40.7234) (-139.3628, -40.7425) (-139.3945, -40.7617) (-139.4262, -40.7812) (-139.4579, -40.8008) (-139.4895, -40.8207) (-139.521, -40.8407) (-139.5525, -40.861) (-139.5839, -40.8814) (-139.6153, -40.9021) (-139.6466, -40.9229) (-139.6778, -40.9439) (-139.709, -40.9651) (-139.7402, -40.9866) (-139.7713, -41.0082) (-139.8023, -41.0299) (-139.8332, -41.0519) (-139.8641, -41.0741) (-139.895, -41.0964) (-139.9196, -41.1145) (-139.9381, -41.1281) (-139.9503, -41.1372) (-139.9565, -41.1417) knots 0 0 0 0 0 0 0.01428571 0.02857143 0.04285714 0.05714286 0.07142857 0.08571429 0.1 0.11428571 0.12857143 0.14285714 0.15714286 0.17142857 0.18571429 0.2 0.21428571 0.22857143 0.24285714 0.25714286 0.27142857 0.28571429 0.3 0.31428571 0.32857143 0.34285714 0.35714286 0.37142857 0.38571429 0.4 0.41428571 0.42857143 0.44285714 0.45714286 0.47142857 0.48571429 0.5 0.51428571 0.52857143 0.54285714 0.55714286 0.57142857 0.58571429 0.6 0.61428571 0.62857143 0.64285714 0.65714286 0.67142857 0.68571429 0.7 0.71428571 0.72857143 0.74285714 0.75714286 0.77142857 0.78571429 0.8 0.81428571 0.82857143 0.84285714 0.85714286 0.87142857 0.88571429 0.9 0.91428571 0.92857143 0.94285714 0.95714286 0.97142857 0.98571429 1 1 1 1 1 1
  arc A53 (-139.9565, -41.1417) -> (-139.8557, -42.0753) centre (-125, -40) ccw
  spline S27 degree 5 poles (-137.4153, -42.6059) (-137.422, -42.6073) (-137.4353, -42.6099) (-137.4554, -42.6132) (-137.4823, -42.6167) (-137.5162, -42.6195) (-137.5502, -42.6213) (-137.5843, -42.6225) (-137.6186, -42.6233) (-137.6528, -42.6239) (-137.6871, -42.6242) (-137.7215, -42.6242) (-137.7559, -42.6238) (-137.7904, -42.6229) (-137.8249, -42.6215) (-137.8595, -42.6196) (-137.8942, -42.6173) (-137.9289, -42.6146) (-137.9636, -42.6117) (-137.9984, -42.6084) (-138.0332, -42.6049) (-138.068, -42.6011) (-138.1029, -42.597) (-138.1378, -42.5926) (-138.1727, -42.5879) (-138.2076, -42.5828) (-138.2426, -42.5774) (-138.2776, -42.5718) (-138.3126, -42.5659) (-138.3476, -42.5598) (-138.3826, -42.5534) (-138.4177, -42.5467) (-138.4527, -42.5398) (-138.4878, -42.5326) (-138.5229, -42.5251) (-138.558, -42.5174) (-138.5931, -42.5095) (-138.6282, -42.5013) (-138.6634, -42.4928) (-138.6985, -42.4842) (-138.7336, -42.4753) (-138.7688, -42.4661) (-138.8039, -42.4567) (-138.8391, -42.4471) (-138.8742, -42.4373) (-138.9094, -42.4272) (-138.9446, -42.4169) (-138.9797, -42.4064) (-139.0149, -42.3957) (-139.05, -42.3847) (-139.0851, -42.3736) (-139.1203, -42.3622) (-139.1554, -42.3506) (-139.1905, -42.3388) (-139.2257, -42.3267) (-139.2608, -42.3145) (-139.2959, -42.302) (-139.331, -42.2894) (-139.3661, -42.2765) (-139.4011, -42.2635) (-139.4362, -42.2502) (-139.4712, -42.2367) (-139.5063, -42.223) (-139.5413, -42.2091) (-139.5763, -42.1951) (-139.6113, -42.1808) (-139.6463, -42.1663) (-139.6812, -42.1516) (-139.7162, -42.1368) (-139.7511, -42.1217) (-139.786, -42.1065) (-139.8139, -42.0941) (-139.8348, -42.0848) (-139.8488, -42.0785) (-139.8557, -42.0753) knots 0 0 0 0 0 0 0.01428571 0.02857143 0.04285714 0.05714286 0.07142857 0.08571429 0.1 0.11428571 0.12857143 0.14285714 0.15714286 0.17142857 0.18571429 0.2 0.21428571 0.22857143 0.24285714 0.25714286 0.27142857 0.28571429 0.3 0.31428571 0.32857143 0.34285714 0.35714286 0.37142857 0.38571429 0.4 0.41428571 0.42857143 0.44285714 0.45714286 0.47142857 0.48571429 0.5 0.51428571 0.52857143 0.54285714 0.55714286 0.57142857 0.58571429 0.6 0.61428571 0.62857143 0.64285714 0.65714286 0.67142857 0.68571429 0.7 0.71428571 0.72857143 0.74285714 0.75714286 0.77142857 0.78571429 0.8 0.81428571 0.82857143 0.84285714 0.85714286 0.87142857 0.88571429 0.9 0.91428571 0.92857143 0.94285714 0.95714286 0.97142857 0.98571429 1 1 1 1 1 1
  line L27 (-137.4153, -42.6059) -> (-136.993, -42.5172)
  arc A54 (-136.4055, -42.884) -> (-136.993, -42.5172) centre (-136.8903, -43.0066) ccw
  arc A55 (-136.4055, -42.884) -> (-136.1806, -43.6604) centre (-125, -40) ccw
  arc A56 (-136.4809, -44.2844) -> (-136.1806, -43.6604) centre (-136.6558, -43.8159) ccw
  line L28 (-136.4809, -44.2844) -> (-136.8853, -44.4353)
  spline S28 degree 5 poles (-136.8853, -44.4353) (-136.8916, -44.4376) (-136.9043, -44.4425) (-136.923, -44.4504) (-136.9476, -44.4619) (-136.9778, -44.4776) (-137.0075, -44.4943) (-137.037, -44.5116) (-137.0663, -44.5292) (-137.0956, -44.547) (-137.1248, -44.5651) (-137.1538, -44.5834) (-137.1827, -44.6022) (-137.2113, -44.6214) (-137.2398, -44.6411) (-137.268, -44.6612) (-137.296, -44.6816) (-137.324, -44.7024) (-137.3517, -44.7235) (-137.3794, -44.7448) (-137.4069, -44.7664) (-137.4343, -44.7882) (-137.4616, -44.8103) (-137.4887, -44.8327) (-137.5156, -44.8554) (-137.5425, -44.8783) (-137.5692, -44.9015) (-137.5957, -44.925) (-137.6222, -44.9487) (-137.6485, -44.9726) (-137.6746, -44.9968) (-137.7007, -45.0211) (-137.7266, -45.0457) (-137.7524, -45.0706) (-137.7781, -45.0956) (-137.8036, -45.1209) (-137.8291, -45.1464) (-137.8544, -45.1721) (-137.8795, -45.198) (-137.9046, -45.2241) (-137.9295, -45.2504) (-137.9543, -45.277) (-137.979, -45.3037) (-138.0036, -45.3306) (-138.0281, -45.3577) (-138.0524, -45.385) (-138.0766, -45.4125) (-138.1007, -45.4402) (-138.1246, -45.468) (-138.1485, -45.4961) (-138.1722, -45.5243) (-138.1958, -45.5527) (-138.2193, -45.5813) (-138.2427, -45.6101) (-138.2659, -45.639) (-138.2891, -45.6681) (-138.3121, -45.6974) (-138.335, -45.7269) (-138.3577, -45.7565) (-138.3804, -45.7863) (-138.4029, -45.8162) (-138.4253, -45.8464) (-138.4476, -45.8767) (-138.4698, -45.9071) (-138.4919, -45.9377) (-138.5138, -45.9685) (-138.5356, -45.9994) (-138.5573, -46.0305) (-138.5789, -46.0618) (-138.6004, -46.0931) (-138.6217, -46.1247) (-138.6387, -46.1501) (-138.6514, -46.1692) (-138.6598, -46.1819) (-138.664, -46.1883) knots 0 0 0 0 0 0 0.01428571 0.02857143 0.04285714 0.05714286 0.07142857 0.08571429 0.1 0.11428571 0.12857143 0.14285714 0.15714286 0.17142857 0.18571429 0.2 0.21428571 0.22857143 0.24285714 0.25714286 0.27142857 0.28571429 0.3 0.31428571 0.32857143 0.34285714 0.35714286 0.37142857 0.38571429 0.4 0.41428571 0.42857143 0.44285714 0.45714286 0.47142857 0.48571429 0.5 0.51428571 0.52857143 0.54285714 0.55714286 0.57142857 0.58571429 0.6 0.61428571 0.62857143 0.64285714 0.65714286 0.67142857 0.68571429 0.7 0.71428571 0.72857143 0.74285714 0.75714286 0.77142857 0.78571429 0.8 0.81428571 0.82857143 0.84285714 0.85714286 0.87142857 0.88571429 0.9 0.91428571 0.92857143 0.94285714 0.95714286 0.97142857 0.98571429 1 1 1 1 1 1
  arc A57 (-138.664, -46.1883) -> (-138.25, -47.0311) centre (-125, -40) ccw
  spline S29 degree 5 poles (-135.7753, -46.695) (-135.7811, -46.6986) (-135.7927, -46.7056) (-135.8104, -46.7156) (-135.8346, -46.728) (-135.8654, -46.7423) (-135.8968, -46.7557) (-135.9285, -46.7684) (-135.9603, -46.7809) (-135.9923, -46.7932) (-136.0245, -46.8052) (-136.0567, -46.817) (-136.0892, -46.8284) (-136.1219, -46.8393) (-136.1549, -46.8498) (-136.1881, -46.8598) (-136.2214, -46.8695) (-136.2549, -46.8789) (-136.2886, -46.888) (-136.3224, -46.8969) (-136.3563, -46.9055) (-136.3903, -46.9138) (-136.4244, -46.9219) (-136.4587, -46.9296) (-136.4932, -46.9371) (-136.5277, -46.9443) (-136.5624, -46.9512) (-136.5972, -46.9579) (-136.6321, -46.9644) (-136.6671, -46.9705) (-136.7022, -46.9765) (-136.7375, -46.9822) (-136.7728, -46.9877) (-136.8082, -46.9929) (-136.8437, -46.9979) (-136.8793, -47.0027) (-136.9151, -47.0073) (-136.9509, -47.0116) (-136.9868, -47.0156) (-137.0228, -47.0195) (-137.0588, -47.0232) (-137.095, -47.0266) (-137.1312, -47.0298) (-137.1675, -47.0328) (-137.2039, -47.0356) (-137.2404, -47.0381) (-137.277, -47.0405) (-137.3136, -47.0426) (-137.3503, -47.0446) (-137.3871, -47.0463) (-137.4239, -47.0478) (-137.4608, -47.0491) (-137.4978, -47.0503) (-137.5349, -47.0512) (-137.572, -47.0519) (-137.6091, -47.0524) (-137.6464, -47.0527) (-137.6837, -47.0528) (-137.7211, -47.0527) (-137.7585, -47.0524) (-137.796, -47.0519) (-137.8335, -47.0513) (-137.8711, -47.0504) (-137.9088, -47.0493) (-137.9465, -47.0481) (-137.9843, -47.0466) (-138.0221, -47.045) (-138.0599, -47.0432) (-138.0979, -47.0411) (-138.1358, -47.0389) (-138.1738, -47.0365) (-138.2043, -47.0345) (-138.2271, -47.0328) (-138.2424, -47.0317) (-138.25, -47.0311) knots 0 0 0 0 0 0 0.01428571 0.02857143 0.04285714 0.05714286 0.07142857 0.08571429 0.1 0.11428571 0.12857143 0.14285714 0.15714286 0.17142857 0.18571429 0.2 0.21428571 0.22857143 0.24285714 0.25714286 0.27142857 0.28571429 0.3 0.31428571 0.32857143 0.34285714 0.35714286 0.37142857 0.38571429 0.4 0.41428571 0.42857143 0.44285714 0.45714286 0.47142857 0.48571429 0.5 0.51428571 0.52857143 0.54285714 0.55714286 0.57142857 0.58571429 0.6 0.61428571 0.62857143 0.64285714 0.65714286 0.67142857 0.68571429 0.7 0.71428571 0.72857143 0.74285714 0.75714286 0.77142857 0.78571429 0.8 0.81428571 0.82857143 0.84285714 0.85714286 0.87142857 0.88571429 0.9 0.91428571 0.92857143 0.94285714 0.95714286 0.97142857 0.98571429 1 1 1 1 1 1
  line L29 (-135.7753, -46.695) -> (-135.4088, -46.4673)
  arc A58 (-134.7313, -46.611) -> (-135.4088, -46.4673) centre (-135.1449, -46.892) ccw
  arc A59 (-134.7313, -46.611) -> (-134.2544, -47.2636) centre (-125, -40) ccw
  arc A60 (-134.3232, -47.9527) -> (-134.2544, -47.2636) centre (-134.6477, -47.5723) ccw
  line L30 (-134.3232, -47.9527) -> (-134.6515, -48.2328)
  spline S30 degree 5 poles (-134.6515, -48.2328) (-134.6567, -48.2372) (-134.6669, -48.2461) (-134.6818, -48.26) (-134.701, -48.2792) (-134.724, -48.3042) (-134.7462, -48.3301) (-134.768, -48.3564) (-134.7896, -48.383) (-134.811, -48.4097) (-134.8322, -48.4367) (-134.8532, -48.4638) (-134.8739, -48.4913) (-134.8943, -48.5192) (-134.9143, -48.5474) (-134.9339, -48.576) (-134.9533, -48.6048) (-134.9724, -48.6339) (-134.9913, -48.6632) (-135.01, -48.6927) (-135.0285, -48.7223) (-135.0468, -48.7522) (-135.0648, -48.7823) (-135.0826, -48.8126) (-135.1002, -48.8432) (-135.1176, -48.8739) (-135.1347, -48.9048) (-135.1517, -48.936) (-135.1684, -48.9673) (-135.1849, -48.9987) (-135.2013, -49.0304) (-135.2174, -49.0622) (-135.2334, -49.0942) (-135.2491, -49.1264) (-135.2647, -49.1587) (-135.28, -49.1912) (-135.2952, -49.2238) (-135.3102, -49.2566) (-135.325, -49.2896) (-135.3396, -49.3227) (-135.354, -49.356) (-135.3683, -49.3894) (-135.3823, -49.4229) (-135.3962, -49.4566) (-135.4099, -49.4904) (-135.4235, -49.5244) (-135.4368, -49.5585) (-135.45, -49.5928) (-135.463, -49.6272) (-135.4758, -49.6617) (-135.4884, -49.6963) (-135.5009, -49.7311) (-135.5132, -49.766) (-135.5253, -49.801) (-135.5372, -49.8361) (-135.549, -49.8714) (-135.5606, -49.9068) (-135.5721, -49.9423) (-135.5833, -49.9779) (-135.5944, -50.0137) (-135.6054, -50.0495) (-135.6161, -50.0855) (-135.6267, -50.1216) (-135.6371, -50.1578) (-135.6474, -50.1941) (-135.6575, -50.2305) (-135.6674, -50.2671) (-135.6772, -50.3037) (-135.6868, -50.3404) (-135.6962, -50.3773) (-135.7054, -50.4142) (-135.7127, -50.4439) (-135.7181, -50.4662) (-135.7217, -50.481) (-135.7234, -50.4885) knots 0 0 0 0 0 0 0.01428571 0.02857143 0.04285714 0.05714286 0.07142857 0.08571429 0.1 0.11428571 0.12857143 0.14285714 0.15714286 0.17142857 0.18571429 0.2 0.21428571 0.22857143 0.24285714 0.25714286 0.27142857 0.28571429 0.3 0.31428571 0.32857143 0.34285714 0.35714286 0.37142857 0.38571429 0.4 0.41428571 0.42857143 0.44285714 0.45714286 0.47142857 0.48571429 0.5 0.51428571 0.52857143 0.54285714 0.55714286 0.57142857 0.58571429 0.6 0.61428571 0.62857143 0.64285714 0.65714286 0.67142857 0.68571429 0.7 0.71428571 0.72857143 0.74285714 0.75714286 0.77142857 0.78571429 0.8 0.81428571 0.82857143 0.84285714 0.85714286 0.87142857 0.88571429 0.9 0.91428571 0.92857143 0.94285714 0.95714286 0.97142857 0.98571429 1 1 1 1 1 1
  arc A61 (-135.7234, -50.4885) -> (-135.0462, -51.1389) centre (-125, -40) ccw
  spline S31 degree 5 poles (-132.8357, -49.9766) (-132.8399, -49.982) (-132.8484, -49.9925) (-132.8616, -50.008) (-132.88, -50.0279) (-132.9041, -50.0519) (-132.9291, -50.0752) (-132.9545, -50.098) (-132.9801, -50.1206) (-133.006, -50.1431) (-133.0321, -50.1654) (-133.0584, -50.1875) (-133.085, -50.2093) (-133.112, -50.2308) (-133.1394, -50.2519) (-133.1671, -50.2727) (-133.1952, -50.2932) (-133.2235, -50.3134) (-133.252, -50.3335) (-133.2807, -50.3534) (-133.3096, -50.3731) (-133.3387, -50.3925) (-133.368, -50.4118) (-133.3976, -50.4308) (-133.4274, -50.4496) (-133.4574, -50.4682) (-133.4876, -50.4866) (-133.5181, -50.5048) (-133.5487, -50.5228) (-133.5794, -50.5406) (-133.6104, -50.5582) (-133.6415, -50.5756) (-133.6729, -50.5928) (-133.7044, -50.6099) (-133.736, -50.6267) (-133.7679, -50.6434) (-133.7999, -50.6599) (-133.8321, -50.6762) (-133.8644, -50.6923) (-133.8969, -50.7082) (-133.9295, -50.724) (-133.9623, -50.7396) (-133.9953, -50.755) (-134.0284, -50.7702) (-134.0616, -50.7853) (-134.095, -50.8001) (-134.1286, -50.8149) (-134.1623, -50.8294) (-134.1961, -50.8438) (-134.2301, -50.858) (-134.2642, -50.872) (-134.2984, -50.8859) (-134.3328, -50.8996) (-134.3673, -50.9131) (-134.4019, -50.9265) (-134.4367, -50.9397) (-134.4716, -50.9527) (-134.5066, -50.9655) (-134.5417, -50.9782) (-134.577, -50.9908) (-134.6124, -51.0031) (-134.6479, -51.0153) (-134.6835, -51.0274) (-134.7193, -51.0393) (-134.7551, -51.051) (-134.7911, -51.0625) (-134.8272, -51.0739) (-134.8634, -51.0852) (-134.8997, -51.0962) (-134.9362, -51.1072) (-134.9727, -51.1179) (-135.002, -51.1264) (-135.0241, -51.1327) (-135.0388, -51.1368) (-135.0462, -51.1389) knots 0 0 0 0 0 0 0.01428571 0.02857143 0.04285714 0.05714286 0.07142857 0.08571429 0.1 0.11428571 0.12857143 0.14285714 0.15714286 0.17142857 0.18571429 0.2 0.21428571 0.22857143 0.24285714 0.25714286 0.27142857 0.28571429 0.3 0.31428571 0.32857143 0.34285714 0.35714286 0.37142857 0.38571429 0.4 0.41428571 0.42857143 0.44285714 0.45714286 0.47142857 0.48571429 0.5 0.51428571 0.52857143 0.54285714 0.55714286 0.57142857 0.58571429 0.6 0.61428571 0.62857143 0.64285714 0.65714286 0.67142857 0.68571429 0.7 0.71428571 0.72857143 0.74285714 0.75714286 0.77142857 0.78571429 0.8 0.81428571 0.82857143 0.84285714 0.85714286 0.87142857 0.88571429 0.9 0.91428571 0.92857143 0.94285714 0.95714286 0.97142857 0.98571429 1 1 1 1 1 1
  line L31 (-132.8357, -49.9766) -> (-132.5691, -49.6372)
  arc A62 (-131.8833, -49.5406) -> (-132.5691, -49.6372) centre (-132.1759, -49.9461) ccw
  arc A63 (-131.8833, -49.5406) -> (-131.212, -49.9907) centre (-125, -40) ccw
  arc A64 (-131.041, -50.6618) -> (-131.212, -49.9907) centre (-131.476, -50.4153) ccw
  line L32 (-131.041, -50.6618) -> (-131.2537, -51.0373)
  spline S32 degree 5 poles (-131.2537, -51.0373) (-131.2571, -51.0432) (-131.2636, -51.0551) (-131.2729, -51.0732) (-131.2843, -51.0978) (-131.2973, -51.1292) (-131.3094, -51.1611) (-131.3209, -51.1933) (-131.332, -51.2256) (-131.343, -51.2581) (-131.3537, -51.2907) (-131.3642, -51.3234) (-131.3743, -51.3563) (-131.3839, -51.3895) (-131.393, -51.4228) (-131.4017, -51.4564) (-131.41, -51.4901) (-131.418, -51.524) (-131.4258, -51.5579) (-131.4333, -51.592) (-131.4405, -51.6263) (-131.4474, -51.6606) (-131.4541, -51.695) (-131.4605, -51.7296) (-131.4666, -51.7643) (-131.4724, -51.7992) (-131.4779, -51.8341) (-131.4832, -51.8691) (-131.4882, -51.9043) (-131.493, -51.9395) (-131.4975, -51.9748) (-131.5018, -52.0103) (-131.5058, -52.0458) (-131.5096, -52.0814) (-131.5132, -52.1171) (-131.5165, -52.1529) (-131.5196, -52.1887) (-131.5225, -52.2247) (-131.5251, -52.2607) (-131.5275, -52.2968) (-131.5297, -52.333) (-131.5316, -52.3693) (-131.5334, -52.4056) (-131.5349, -52.442) (-131.5362, -52.4785) (-131.5373, -52.5151) (-131.5382, -52.5517) (-131.5388, -52.5884) (-131.5393, -52.6251) (-131.5395, -52.6619) (-131.5396, -52.6988) (-131.5394, -52.7357) (-131.539, -52.7727) (-131.5384, -52.8098) (-131.5376, -52.8469) (-131.5366, -52.8841) (-131.5354, -52.9213) (-131.534, -52.9586) (-131.5324, -52.9959) (-131.5306, -53.0333) (-131.5286, -53.0707) (-131.5264, -53.1082) (-131.524, -53.1458) (-131.5215, -53.1833) (-131.5187, -53.221) (-131.5157, -53.2586) (-131.5125, -53.2964) (-131.5092, -53.3341) (-131.5056, -53.3719) (-131.5019, -53.4098) (-131.4979, -53.4477) (-131.4947, -53.478) (-131.4921, -53.5008) (-131.4903, -53.516) (-131.4895, -53.5236) knots 0 0 0 0 0 0 0.01428571 0.02857143 0.04285714 0.05714286 0.07142857 0.08571429 0.1 0.11428571 0.12857143 0.14285714 0.15714286 0.17142857 0.18571429 0.2 0.21428571 0.22857143 0.24285714 0.25714286 0.27142857 0.28571429 0.3 0.31428571 0.32857143 0.34285714 0.35714286 0.37142857 0.38571429 0.4 0.41428571 0.42857143 0.44285714 0.45714286 0.47142857 0.48571429 0.5 0.51428571 0.52857143 0.54285714 0.55714286 0.57142857 0.58571429 0.6 0.61428571 0.62857143 0.64285714 0.65714286 0.67142857 0.68571429 0.7 0.71428571 0.72857143 0.74285714 0.75714286 0.77142857 0.78571429 0.8 0.81428571 0.82857143 0.84285714 0.85714286 0.87142857 0.88571429 0.9 0.91428571 0.92857143 0.94285714 0.95714286 0.97142857 0.98571429 1 1 1 1 1 1
  arc A65 (-131.4895, -53.5236) -> (-130.6306, -53.9031) centre (-125, -40) ccw